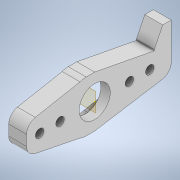
# Autodesk Inventor part: ServoHornAdapter
Saved by Autodesk Inventor 2020 (Build 240168000, 168)
## iProperties
Created: 2020-06-08
Part Number: ServoHornAdapter
Material: Generic
Document SubType Name: Modeling
Designer: Brandon
Density: 1 g/cm^3
Appearance: Default
Author: Brandon
Autodesk Inventor part; units mm, degrees
ref_plane "YZ Plane" through (0, 0, 0) normal (1, 0, 0) x (0, 1, 0)
ref_plane "XZ Plane" through (0, 0, 0) normal (0, 1, 0) x (-1, 0, 0)
ref_plane "XY Plane" through (0, 0, 0) normal (0, 0, 1) x (1, 0, 0)
sketch "Sketch1" plane through (0, 0, 0) normal (1, 0, 0) x (0, 1, 0)
  circle A0 centre (0, 0) radius 3.0734
  line L0 (7.62, 7.62) -> (-7.62, 7.62)
  line L1 (-7.62, 7.62) -> (-7.62, -22.86)
  line L2 (-7.62, -22.86) -> (7.62, -22.86)
  line L3 (7.62, -22.86) -> (7.62, 7.62)
  line L4 (-7.62, -22.86) -> (9.652, -22.86)
  line L5 (9.652, -22.86) -> (9.652, -17.78)
  line L6 (9.652, -17.78) -> (-7.62, -17.78)
  line L7 (-7.62, -17.78) -> (-7.62, -22.86)
  line L8 (7.62, -17.78) -> (4.2265, -17.78)
  line L9 (4.2265, -17.78) -> (4.2265, -10.16)
  line L10 (4.2265, -10.16) -> (7.62, -10.16)
  line L11 (7.62, -10.16) -> (7.62, -17.78)
  arc A1 (4.2265, -12.1082) -> (4.2265, -17.78) centre (8.1105, -14.9441) ccw
  line L12 (4.2265, -12.1082) -> (5.6507, -10.16)
  line L13 (4.2265, -17.78) -> (7.62, 0)
  point P0 (7.62, -17.78)
  point P1 (7.62, -22.86)
  point P2 (7.62, -10.16)
  point P3 (7.62, -10.16)
  point P4 (4.2265, -12.1082)
  dimension "d0" = 6.1468
  dimension "d1" = 7.62
  dimension "d2" = 7.62
  dimension "d3" = 7.62
  dimension "d4" = 22.86
  dimension "d5" = 5.08
  dimension "d6" = 2.032
  dimension "d38" = 7.62
  constraints: 28 end point, 6 parallel, 5 point on line, 3 horizontal, 3 perpendicular, 2 centre point, 2 point on circle, 1 coincident
  measures "d0" diameter of A0
  measures "d1" distance from line of point (0, 0) L3
  measures "d2" distance from line of point (0, 0) L1
  measures "d3" distance from line of point (0, 0) L0
  measures "d4" distance from line of point (0, 0) L2
  measures "d5" distance of L4.end L5.end
  measures "d6" distance between parallel lines of L3 L5
  measures "d38" distance of L8.end L9.end
extrude "Extrusion1" add sketch "Sketch1" along normal blind 5.334 contours L3 L13 L10 L9 A1 L6 L1 L0 | L6 L3 L2 L1 | L13 L9 L12 L10 | A1 L9 | L6 L5 L4 L3 | L12 L9 L10
sketch "Sketch2" plane through (0, 0, 0) normal (-1, 0, 0) x (0, 0, 1)
  circle A0 centre (0, 0) radius 4.6482
  circle A1 centre (0, 0) radius 10.1706
  dimension "d9" = 9.2964
  constraints: 2 centre point, 2 coincident
  measures "d9" diameter of A0
extrude "Extrusion2" cut sketch "Sketch2" against normal blind 5.334 contours A0
fillet "Fillet1" radius 5.08 3 edges at (2.667, -7.62, -22.86) (2.667, 7.62, 7.62) (2.667, -7.62, 7.62)
sketch "Sketch3" plane through (5.334, 0, 0) normal (1, 0, 0) x (0, 0, -1)
  point P0 (0, 0)
sketch "Sketch7" plane through (0, 0, 0) normal (-1, 0, 0) x (0, 0, 1)
  arc A0 (-2.1195, -5.9858) -> (-2.1254, 5.9838) centre (0, 0) ccw
  line L0 (0, 0) -> (-16.4465, 0)
  arc A1 (-16.4465, 3.175) -> (-17.6024, -2.9571) centre (-16.4465, 0) ccw
  line L1 (-0.2923, 6.3433) -> (-16.4465, 3.175)
  circle A2 centre (-16.4465, 0) radius 3.175
  line L2 (-16.4465, -3.175) -> (-0.2923, -6.3433)
  point P0 (-0.2923, -6.3433)
  point P1 (-17.6024, -2.9571)
  dimension "d33" = 12.7
  dimension "d34" = 16.4465
  dimension "d35" = 6.35
  dimension "d54" = 0
  constraints: 7 point on circle, 6 end point, 3 coincident, 2 centre point, 1 horizontal, 1 point on line, 4 other
  measures "d33" diameter of A0
  measures "d34" distance of L0.start L0.end
  measures "d35" diameter of A1
  measures "d54" horizontal distance of A1.centre L1.end
extrude "Extrusion6" cut sketch "Sketch7" against normal blind 2.54 contours L2 A2 L1 A0 | A2 A1
sketch "Sketch8" plane through (2.54, 0, 0) normal (-1, 0, 0) x (0, 0, 1)
  arc A0 (-16.4465, 3.175) -> (-16.4465, -3.175) centre (-16.4465, 0) ccw projected
  line L0 (0, 0) -> (-16.4465, 0)
  circle A1 centre (-16.4465, 0) radius 1.27
  point P0 (-17.7165, -3.175)
  dimension "d39" = 2.54
  dimension "d46" = 16.4465
  constraints: 2 end point, 1 centre point, 1 coincident, 1 horizontal
  measures "d39" diameter of A1
  measures "d46" distance of L0.start L0.end
extrude "Extrusion7" cut sketch "Sketch8" against normal blind 5.334
sketch "Sketch9" plane through (0, 0, 0) normal (-1, 0, 0) x (0, 0, 1)
  line L0 (2.54, -7.62) -> (-17.78, -7.62) projected
  line L1 (0, -7.62) -> (-22.6598, -3.952)
  arc A0 (-22.86, -2.54) -> (-17.78, -7.62) centre (-17.78, -2.54) ccw projected
  point P0 (0, 0)
  constraints: 2 end point, 1 point on circle, 1 point on line
extrude "Extrusion8" cut sketch "Sketch9" against normal blind 5.334
fillet "Fillet2" radius 3.175 1 edges at (2.667, -3.952, -22.6598)
ref_plane "Work Plane1" through (0, -2.54, 0) normal (0, 0, 1) x (1, 0, 0)
mirror "Mirror1" about plane through (0, -2.54, 0) normal (0, 0, 1) of "Extrusion6"
chamfer "Chamfer3" distance 2.54 distance2 5.08 1 edges at (2.667, 9.652, -17.78) measured on face at (1.778, 9.652, -21.1667)
sketch "Sketch10" plane through (2.54, 0, 0) normal (-1, 0, 0) x (0, 0, 1)
  circle A0 centre (-10.3505, 0) radius 1.27
  circle A1 centre (-16.4465, 0) radius 1.27 projected
  point P0 (0, 0)
  dimension "d50" = 2.54
  dimension "d51" = 6.096
  constraints: 1 centre point
  measures "d50" diameter of A0
  measures "d51" distance of A0.centre A1.centre
extrude "Extrusion9" cut sketch "Sketch10" against normal blind 5.334 contours A0
sketch "Sketch11" plane through (0, 0, 0) normal (-1, 0, 0) x (0, 0, 1)
  arc A0 (6.9654, 5.0345) -> (2.54, 7.62) centre (2.54, 2.54) ccw projected
  line L0 (2.54, 7.62) -> (20.32, 4.2879)
  line L1 (20.32, 4.2879) -> (20.32, -4.0399)
  line L2 (20.32, -4.0399) -> (2.54, -7.62)
  arc A1 (2.54, -7.62) -> (6.9654, -5.0345) centre (2.54, -2.54) ccw projected
  line L3 (0, 13.2262) -> (0, -11.7932) projected
  line L4 (0, 7.62) -> (2.54, 7.62) projected
  line L5 (2.54, -7.3934) -> (2.54, -7.62)
  line L6 (2.54, 5.3798) -> (5.1026, 5.3798)
  line L7 (5.1026, 5.3798) -> (5.1026, -5.0345)
  line L8 (5.1026, -5.0345) -> (2.54, -5.0345)
  line L9 (2.54, 7.62) -> (2.54, 5.3798)
  line L10 (2.54, -5.0345) -> (2.54, -7.3934)
  point P0 (0, 0)
  point P1 (2.54, -7.62)
  point P2 (4.5061, -7.2241)
  dimension "d56" = 0
  dimension "d57" = 20.32
  constraints: 18 end point, 3 vertical, 2 point on circle, 1 horizontal, 1 parallel, 1 perpendicular
  measures "d56" distance of L4.end L0.start
  measures "d57" distance between parallel lines of L1 L3
extrude "Extrusion10" add sketch "Sketch11" against normal blind 5.334 contours L0 L1 L2 L5 L10 L8 L7 L6 L9
mirror "Mirror2" about plane through (0, -2.54, 0) normal (0, 0, 1) of "Extrusion6", "Extrusion7", "Extrusion9"
fillet "Fillet3" radius 3.175 2 edges at (2.667, 4.2879, 20.32) (2.667, -4.0399, 20.32)
body "Solid1"
